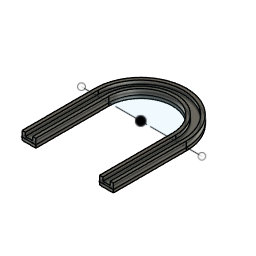
supporter for rotating disc (Autodesk Fusion 360 design; units mm, degrees)
Autodesk Fusion 360 part; units mm, degrees
sketch "Sketch1" plane through (0, 0, 0) normal (0, 0, 1) x (1, 0, 0)
  line L0 (-65, 0) -> (67.0686, 0)
  line L1 (-35, 0) -> (-35, -80)
  line L2 (-50, 0) -> (-50, -80)
  line L3 (35, 0) -> (35, -80)
  line L4 (50, 0) -> (50, -80)
  line L5 (35, -80) -> (50, -80)
  line L6 (-50, -80) -> (-35, -80)
  arc A0 (35, 0) -> (-35, 0) centre (0, 0) ccw
  arc A1 (50, 0) -> (-50, 0) centre (0, 0) ccw
  arc A2 (38.5, 0) -> (-38.5, 0) centre (0, 0) ccw
  arc A3 (46.5, 0) -> (-46.5, 0) centre (0, 0) ccw
  line L7 (-38.5, 0) -> (-38.5, -80)
  line L8 (-46.5, 0) -> (-46.5, -80)
  line L9 (38.5, 0) -> (38.5, -80)
  line L10 (46.5, 0) -> (46.5, -80)
  dimension "d1" = 70
  dimension "d2" = 100
  dimension "d3" = 80
  dimension "d4" = 80
  dimension "d5" = 80
  dimension "d8" = 77
  dimension "d9" = 93
  constraint coincident A0.centre A1.centre
  constraint horizontal L0
  constraint coincident L0 L1.start
  constraint tangent L1 A0
  constraint perpendicular L0 L1
  constraint coincident L0 L2.start
  constraint tangent L2 A1
  constraint coincident L0 L3.start
  constraint tangent L3 A0
  constraint coincident L0 L4.start
  constraint tangent L4 A1
  constraint perpendicular L4 L5
  constraint concentric A0 A3
  constraint coincident L0 A2.end
  constraint coincident L0 A2.start
  constraint coincident L0 A3.end
  constraint coincident L0 A3.start
  constraint coincident L6 L7.end
  constraint tangent A2 L7
  constraint coincident L6 L8.end
  constraint tangent A3 L8
  constraint coincident L5 L9.end
  constraint tangent A2 L9
  constraint coincident L5 L10.end
  constraint tangent A3 L10
  measures "d1" diameter of A0
  measures "d2" diameter of A1
  measures "d3" distance of L1.start L1.end
  measures "d4" distance of L2.start L2.end
  measures "d5" distance of L4.start L4.end
  measures "d8" diameter of A2
  measures "d9" diameter of A3
extrude "Extrude2" add sketch "Sketch1" along normal blind 6 contours L0 A1 A3 | L0 L2 L6 L8 | L0 L4 L5 L10 | L0 A0 A2 | L0 L1 L6 L7 | L0 L3 L5 L9 makes body 1 at (36.1667, -53.3333, 0) makes body 2 at (-47.6667, -53.3333, 0)
extrude "Extrude3" add sketch "Sketch1" along normal blind 2 separate body contours L0 A2 A3 | L0 L6 L7 L8 | L0 L5 L9 L10 makes body 3
extrude "Extrude4" add sketch "Sketch1" against normal blind 3.3 contours L0 A1 A3 | L0 L2 L6 L8 | L0 A2 A3 | L0 L6 L7 L8 | L0 L4 L5 L10 | L0 A0 A2 | L0 L1 L6 L7 | L0 L5 L9 L10 | L0 L3 L5 L9 bodies 1 2 3
